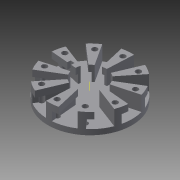
# Autodesk Inventor part: male bayonet connector 12
Saved by Autodesk Inventor 2015 (Build 190159000, 159)
## iProperties
Created: 2014-06-11
Part Number: male bayonet connector 12
Material: Generic
Document SubType Name: Modeling
Designer: ericd_000
Density: 1 g/cm^3
Appearance: Default
Author: ericd_000
Autodesk Inventor part; units mm, degrees
ref_plane "YZ Plane" through (0, 0, 0) normal (1, 0, 0) x (0, 1, 0)
ref_plane "XZ Plane" through (0, 0, 0) normal (0, 1, 0) x (-1, 0, 0)
ref_plane "XY Plane" through (0, 0, 0) normal (0, 0, 1) x (1, 0, 0)
sketch "Sketch19" plane through (0, 0, 0) normal (0, 0, 1) x (1, 0, 0)
  circle A0 centre (0, 0) radius 39.5
  dimension "d94" = 79
  constraints: 1 centre point, 1 coincident
  measures "d94" diameter of A0
extrude "Extrusion20" add sketch "Sketch19" along normal blind 5
sketch "Sketch21" plane through (0, 0, 5) normal (0, 0, 1) x (1, 0, 0)
  point P0 (0, 0)
sketch "Sketch23" plane through (0, 0, 5) normal (0, 0, 1) x (1, 0, 0)
  line L0 (0, 0) -> (20.2843, 33.8939) construction
  circle A0 centre (0, 0) radius 39.5 construction
  line L1 (0, 0) -> (24.804, 30.7411) construction
  circle A1 centre (0, 0) radius 39.5 construction
  line L2 (24.804, 30.7411) -> (9.4735, 11.7411)
  line L3 (9.4735, 11.7411) -> (7.6719, 12.8193)
  line L4 (7.6719, 12.8193) -> (20.2843, 33.8939)
  arc A2 (24.804, 30.7411) -> (20.2843, 33.8939) centre (0, 0) ccw
  dimension "d105" = 172
  dimension "d106" = 19
  constraints: 10 end point, 2 collinear, 2 point on circle, 1 centre point, 1 perpendicular, 5 other
  measures "d105" angle of L0 L1
  measures "d106" vertical distance of L1.end L2.end
extrude "Extrusion21" add sketch "Sketch23" along normal blind 14
sketch "Sketch26" plane through (7.6719, 12.8193, 5) normal (-0.8580744, 0.5135254, 0) x (0, 0, 1)
  line L0 (14, 24.5604) -> (14, 0)
  line L1 (14, 24.5604) -> (8, 24.5604)
  line L2 (0, 24.5604) -> (14, 24.5604) projected
  line L3 (0, 0) -> (14, 0) projected
  line L4 (8, 0) -> (14, 0)
  line L5 (8, 24.5604) -> (8, 0)
  line L6 (-8.8, -14.9396) -> (17.8, -14.9396) projected
  point P0 (-5, -14.9396)
  dimension "d122" = 6
  dimension "d123" = 6
  constraints: 8 end point, 2 point on line, 1 collinear, 1 vertical
  measures "d122" distance of L0.start L1.end
  measures "d123" distance of L4.start L0.end
revolve "Revolution2" add sketch "Sketch26" angle 8 about axis through (0, 0, 5) along (0, 0, 1)
sketch "Sketch25" plane through (0, 0, 19) normal (0, 0, 1) x (1, 0, 0)
  circle A0 centre (17.7275, 27.8341) radius 2.5
  line L0 (17.7275, 27.8341) -> (0, 0) construction
  line L1 (5.8131, 13.7622) -> (15.3697, 36.3871) projected
  dimension "d112" = 5
  dimension "d116" = 33
  dimension "d125" = 5.5
  constraints: 2 end point, 1 centre point
  measures "d112" diameter of A0
  measures "d116" distance of L0.start L0.end
  measures "d125" distance from line of L0.start L1
extrude "Extrusion22" cut sketch "Sketch25" against normal through all
sketch "Sketch27" plane through (0, 0, 19) normal (0, 0, 1) x (1, 0, 0)
  line L0 (7.6719, 12.8193) -> (9.4735, 11.7411) projected
  line L1 (7.6719, 12.8193) -> (5.8131, 13.7622)
  line L2 (5.8131, 13.7622) -> (19.3663, 45.8487)
  line L3 (5.8131, 13.7622) -> (15.3697, 36.3871) projected
  line L4 (19.3663, 45.8487) -> (7.4433, 12.9352)
  point P0 (0, 0)
  constraints: 7 end point, 2 point on line
extrude "Extrusion23" [suppressed]
pattern_circular "Circular Pattern2" count 10 over 360 about axis through (0, 0, 5) along (0, 0, 1) of "Extrusion21", "Revolution2", "Extrusion22"
sketch "Sketch29" plane through (0, 0, 5) normal (0, 0, 1) x (1, 0, 0)
  circle A0 centre (0, 0) radius 59
  line L0 (0, 0) -> (-36.9013, 14.0905)
  line L1 (0, 0) -> (-38.5032, 8.8177)
  line L2 (-14.5626, 3.335) -> (-38.5032, 8.8177) projected
  arc A1 (-20.2843, -33.8939) -> (-1.9977, -39.4495) centre (0, 0) ccw projected
  point P0 (-34.4215, 7.8829)
  dimension "d135" = 118
  constraints: 4 end point, 1 centre point, 1 coincident, 1 collinear, 1 concentric
  measures "d135" diameter of A0
extrude "Extrusion26" [suppressed]
sketch "Sketch30" plane through (0, 0, 5) normal (0, 0, -1) x (-1, 0, 0)
  line L0 (-109.7485, 105.489) -> (97.8298, 105.489)
  line L1 (97.8298, 105.489) -> (97.8298, -69.3705)
  line L2 (97.8298, -69.3705) -> (-109.7485, -69.3705)
  line L3 (-109.7485, -69.3705) -> (-109.7485, 105.489)
  line L4 (32.0383, -2.0031) -> (28.8173, 14.5454)
  line L5 (28.8173, 14.5454) -> (71.7406, 33.7946)
  line L6 (71.7406, 33.7946) -> (71.7406, -3.6949)
  line L7 (71.7406, -3.6949) -> (32.0383, -2.0031)
  point P0 (0, 0)
  constraints: 16 end point, 2 parallel, 1 horizontal, 1 perpendicular, 1 vertical
extrude "Extrusion27" [suppressed]
sketch "Sketch31" plane through (-39.3557, 3.3732, 19) normal (0, 0, 1) x (0.9963469, -0.0853985, 0)
  line L0 (16, 0) -> (20, 0)
  line L1 (20, 0) -> (20, 3)
  line L2 (20, 3) -> (16, 3)
  line L3 (16, 3) -> (16, 0)
  line L4 (24.5604, 0) -> (0, 0) projected
  point P0 (39.5, 0)
  point P1 (24.7502, 0)
  dimension "d148" = 16
  dimension "d149" = 4
  dimension "d150" = 3
  constraints: 8 end point, 2 parallel, 1 collinear, 1 horizontal, 1 perpendicular
  measures "d148" distance from line of L3 L4.end
  measures "d149" distance of L1.end L2.end
  measures "d150" distance of L0.end L1.end
extrude "Extrusion28" cut sketch "Sketch31" against normal up to surface (6 mm away)
body "Solid2"
